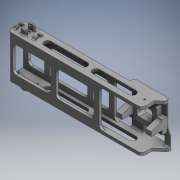
# Autodesk Inventor part: Arm Bottom Left
Saved by Autodesk Inventor 2020.5 (Build 245400000, 400)
## iProperties
Created: 2023-03-21
Part Number: Arm Bottom Left
Material: Generic
Document SubType Name: Modeling
Designer: Wes
Density: 1 g/cm^3
Appearance: Default
Author: Wes
Autodesk Inventor part; units mm, degrees
ref_plane "YZ Plane" through (0, 0, 0) normal (1, 0, 0) x (0, 1, 0)
ref_plane "XZ Plane" through (0, 0, 0) normal (0, 1, 0) x (-1, 0, 0)
ref_plane "XY Plane" through (0, 0, 0) normal (0, 0, 1) x (1, 0, 0)
sketch "Base" plane through (0, 0, 0) normal (0, 0, 1) x (1, 0, 0)
  line L0 (0, 0) -> (-30, 0)
  line L1 (-30, 0) -> (-30, 230)
  line L2 (-30, 230) -> (0, 230)
  line L3 (0, 230) -> (0, 0)
  dimension "d0" = 30
  dimension "d1" = 230
  constraints: 8 end point, 2 parallel, 1 horizontal, 1 perpendicular
  measures "d0" distance of L1.end L2.end
  measures "d1" distance of L0.end L1.end
extrude "Extrusion1" add sketch "Base" along normal blind 5
sketch "Axle Screw Countersink" plane through (0, 0, 5) normal (0, 0, 1) x (1, 0, 0)
  line L0 (-15, 0) -> (-15, 20) construction
  circle A0 centre (-15, 20) radius 3.15
  dimension "d4" = 20
  dimension "d58" = 6.3
  constraints: 2 end point, 1 centre point, 1 coincident, 1 vertical
  measures "d4" distance of L0.start L0.end
  measures "d58" diameter of A0
extrude "Extrusion2" cut sketch "Axle Screw Countersink" against normal blind 1.2
sketch "Motor Arm Center Fitting" plane through (0, 0, 5) normal (0, 0, 1) x (1, 0, 0)
  line L0 (-19.393, 15.95) -> (-19.393, 24.05) construction
  arc A0 (-19.393, 24.05) -> (-19.393, 15.95) centre (-15, 20) ccw
  line L1 (-19.393, 15.95) -> (-21.231, 14.2554)
  line L2 (-19.393, 24.05) -> (-21.231, 25.7446)
  line L3 (-15, 8.3504) -> (-15, 30.6989) construction
  arc A1 (-21.231, 25.7446) -> (-21.231, 14.2554) centre (-15, 20) ccw
  line L4 (-10.607, 15.95) -> (-10.607, 24.05) construction
  line L5 (-10.607, 15.95) -> (-19.393, 15.95) construction
  arc A2 (-10.607, 15.95) -> (-10.607, 24.05) centre (-15, 20) ccw
  line L6 (-10.607, 15.95) -> (-8.769, 14.2554)
  line L7 (-10.607, 24.05) -> (-8.769, 25.7446)
  arc A3 (-8.769, 14.2554) -> (-8.769, 25.7446) centre (-15, 20) ccw
  circle A4 centre (-15, 20) radius 5.975 construction
  point P0 (0, 0)
  point P1 (-15, 20)
  dimension "d18" = 11.95
  dimension "d19" = 8.1
  dimension "d20" = 8.1
  dimension "d21" = 2.5
  dimension "d22" = 2.5
  constraints: 16 end point, 12 point on circle, 5 centre point, 2 line through centre, 2 symmetric about line, 2 vertical, 1 concentric, 1 perpendicular, 2 other
  measures "d18" diameter of A4
  measures "d19" distance of L5.start L4.end
  measures "d20" distance of L5.end L0.end
  measures "d21" distance of L5.end L1.end
  measures "d22" distance of L0.end L2.end
extrude "Extrusion3" add sketch "Motor Arm Center Fitting" along normal blind 5
sketch "Motor Rotation Support" plane through (0, 0, 10) normal (0, 0, 1) x (1, 0, 0)
  line L0 (-20.975, 20) -> (-21.775, 20) construction
  circle A0 centre (-15, 20) radius 6.775 construction
  arc A1 (-19.9811, 24.5923) -> (-19.9811, 15.4077) centre (-15, 20) ccw
  line L1 (-21.775, 20) -> (-23.775, 20) construction
  circle A2 centre (-15, 20) radius 8.775 construction
  arc A3 (-21.4516, 25.9479) -> (-21.4516, 14.0521) centre (-15, 20) ccw
  line L2 (-21.4516, 14.0521) -> (-19.9811, 15.4077)
  line L3 (-19.9811, 24.5923) -> (-21.4516, 25.9479)
  line L4 (-15, 8.5295) -> (-15, 32.0479) construction
  line L5 (-8.5484, 14.0521) -> (-10.0189, 15.4077)
  arc A4 (-8.5484, 14.0521) -> (-8.5484, 25.9479) centre (-15, 20) ccw
  arc A5 (-10.0189, 15.4077) -> (-10.0189, 24.5923) centre (-15, 20) ccw
  line L6 (-10.0189, 24.5923) -> (-8.5484, 25.9479)
  point P0 (0, 0)
  point P1 (-21.231, 14.2554)
  point P2 (-21.231, 25.7446)
  dimension "d25" = 0.8
  dimension "d26" = 2
  constraints: 16 point on circle, 14 end point, 6 centre point, 4 symmetric about line, 2 coincident, 2 horizontal, 1 concentric, 1 vertical, 2 other
  measures "d25" distance of L0.start L0.end
  measures "d26" distance of L0.end L1.end
extrude "Extrusion4" add sketch "Motor Rotation Support" along normal blind 3.35
sketch "Motor Arm Screw Holes" plane through (0, 0, 5) normal (0, 0, 1) x (1, 0, 0)
  line L0 (-15, 20) -> (-15, 37.1) construction
  line L1 (-15, 20) -> (-15, 2.9) construction
  line L2 (-15, 20) -> (-15, 4.2) construction
  line L3 (-15, 20) -> (-15, 35.8) construction
  line L4 (-15, 4.2) -> (-15, 2.9) construction
  line L5 (-15, 35.8) -> (-15, 37.1) construction
  circle A0 centre (-15, 36.45) radius 1.175
  circle A1 centre (-15, 3.55) radius 1.175
  point P0 (0, 0)
  dimension "d59" = 34.2
  dimension "d60" = 31.6
  dimension "d61" = 2.35
  dimension "d62" = 2.35
  constraints: 12 end point, 3 vertical, 2 centre point, 2 midpoint, 2 point on line, 1 coincident, 1 collinear
  measures "d59" distance of L0.end L1.end
  measures "d60" distance of L3.end L2.end
  measures "d61" diameter of A0
  measures "d62" diameter of A1
extrude "Extrusion5" cut sketch "Motor Arm Screw Holes" against normal through all
sketch "Motor Arm Support" plane through (0, 0, 5) normal (0, 0, 1) x (1, 0, 0)
  line L0 (-15, 2.375) -> (-15, 6.875) construction
  line L1 (-15, 6.875) -> (-11.875, 6.875) construction
  line L2 (-15, 6.875) -> (-18.125, 6.875) construction
  line L3 (-15, 3.55) -> (-12.2, 3.55) construction
  line L4 (-15, 3.55) -> (-12.2, 3.55) construction
  line L5 (-15, 3.55) -> (-17.8, 3.55) construction
  line L6 (-15, 3.55) -> (-12.2, 3.55) construction
  line L7 (-18.125, 6.875) -> (-17.8, 3.55)
  line L8 (-17.8, 3.55) -> (-19.7905, 3.3554)
  line L9 (-19.7905, 3.3554) -> (-20.1155, 6.6804)
  line L10 (-20.1155, 6.6804) -> (-18.125, 6.875)
  line L11 (-11.875, 6.875) -> (-12.2, 3.55)
  line L12 (-12.2, 3.55) -> (-10.2095, 3.3554)
  line L13 (-9.8845, 6.6804) -> (-11.875, 6.875)
  line L14 (-10.2095, 3.3554) -> (-9.8845, 6.6804)
  line L15 (-17.8, 3.55) -> (-17.6054, 1.5595)
  line L16 (-17.6054, 1.5595) -> (-19.596, 1.3649)
  line L17 (-19.596, 1.3649) -> (-19.7905, 3.3554)
  line L18 (-12.2, 3.55) -> (-12.3946, 1.5595)
  line L19 (-12.3946, 1.5595) -> (-10.404, 1.3649)
  line L20 (-10.404, 1.3649) -> (-10.2095, 3.3554)
  arc A0 (-10.607, 15.95) -> (-10.607, 24.05) centre (-15, 20) ccw construction
  line L21 (-9.025, 20) -> (-20.975, 20) construction
  arc A1 (-19.393, 24.05) -> (-19.393, 15.95) centre (-15, 20) ccw construction
  line L22 (-15, 33.125) -> (-11.875, 33.125) construction
  line L23 (-15, 33.125) -> (-18.125, 33.125) construction
  line L24 (-11.875, 33.125) -> (-12.2, 36.45)
  line L25 (-10.2095, 36.6446) -> (-9.8845, 33.3196)
  line L26 (-9.8845, 33.3196) -> (-11.875, 33.125)
  line L27 (-18.125, 33.125) -> (-17.8, 36.45)
  line L28 (-19.7905, 36.6446) -> (-20.1155, 33.3196)
  line L29 (-20.1155, 33.3196) -> (-18.125, 33.125)
  line L30 (-17.8, 36.45) -> (-19.7905, 36.6446)
  line L31 (-15, 37.625) -> (-15, 33.125) construction
  line L32 (-15, 36.45) -> (-12.2, 36.45) construction
  line L33 (-15, 36.45) -> (-12.2, 36.45) construction
  line L34 (-15, 36.45) -> (-17.8, 36.45) construction
  line L35 (-15, 36.45) -> (-12.2, 36.45) construction
  line L36 (-19.596, 38.6351) -> (-19.7905, 36.6446)
  line L37 (-17.6054, 38.4405) -> (-19.596, 38.6351)
  line L38 (-17.8, 36.45) -> (-17.6054, 38.4405)
  line L39 (-12.2, 36.45) -> (-12.3946, 38.4405)
  line L40 (-12.2, 36.45) -> (-10.2095, 36.6446)
  line L41 (-10.404, 38.6351) -> (-10.2095, 36.6446)
  line L42 (-12.3946, 38.4405) -> (-10.404, 38.6351)
  point P0 (0, 0)
  dimension "d63" = 4.5
  dimension "d64" = 6.25
  dimension "d65" = 5.6
  dimension "d66" = 2
  dimension "d67" = 2
  constraints: 86 end point, 22 symmetric about line, 7 horizontal, 5 perpendicular, 2 collinear, 2 point on circle, 1 vertical
  measures "d63" distance of L0.start L1.start
  measures "d64" distance of L2.end L1.end
  measures "d65" distance of L7.end L3.end
  measures "d66" distance of L7.end L9.start
  measures "d67" distance of L7.end L16.start
extrude "Extrusion6" add sketch "Motor Arm Support" along normal blind 3
draft "FaceDraft1" angle 28 pull direction (0, 0, 1) faces at (-10.2309, 3.1368, 6) (-10.0577, 35.0914, 6) fixed edges at (-10.1443, 4.0227, 8) (-10.1443, 35.9773, 8)
draft "FaceDraft2" angle 28 pull direction (0, 0, 1) faces at (-19.9423, 4.9086, 6) (-19.7691, 36.8632, 6) fixed edges at (-19.8557, 4.0227, 8) (-19.8557, 35.9773, 8)
sketch "Axle Hole" plane through (0, 0, 5) normal (0, 0, 1) x (1, 0, 0)
  line L0 (0, 230) -> (-30, 230) construction
  line L1 (-15, 230) -> (-15, 220) construction
  circle A0 centre (-15, 220) radius 1.5
  point P0 (0, 0)
  dimension "d73" = 10
  dimension "d74" = 3
  constraints: 2 end point, 1 centre point, 1 coincident, 1 midpoint, 1 vertical
  measures "d73" distance of L1.start L1.end
  measures "d74" diameter of A0
extrude "Extrusion7" cut sketch "Axle Hole" against normal through all
sketch "Motor Backplate Offset" plane through (0, 0, 0) normal (0, 0, -1) x (-1, 0, 0)
  circle A0 centre (15, 220) radius 1.5 construction
  line L0 (15, 220) -> (15, 180) construction
  line L1 (15, 220) -> (15, 240) construction
  line L2 (30, 240) -> (33.5, 240)
  line L3 (33.5, 240) -> (33.5, 180)
  line L4 (33.5, 180) -> (30, 180)
  line L5 (30, 180) -> (30, 240)
  point P0 (0, 0)
  dimension "d77" = 40
  dimension "d78" = 20
  dimension "d83" = 3.5
  dimension "d84" = 60
  constraints: 12 end point, 2 parallel, 2 vertical, 1 horizontal, 1 perpendicular
  measures "d77" distance of L0.start L0.end
  measures "d78" distance of L0.start L1.end
  measures "d83" distance of L3.end L4.end
  measures "d84" distance of L0.end L1.end
extrude "Extrusion8" add sketch "Motor Backplate Offset" against normal up to surface (5 mm away)
sketch "Motor Backplate" plane through (0, 0, 0) normal (0, 0, -1) x (-1, 0, 0)
  line L0 (33.5, 180) -> (33.5, 240) projected
  line L1 (33.5, 240) -> (37.5, 240)
  line L2 (37.5, 240) -> (37.5, 180)
  line L3 (37.5, 180) -> (33.5, 180)
  line L4 (33.5, 180) -> (33.5, 240)
  point P0 (0, 0)
  dimension "d85" = 4
  constraints: 8 end point, 2 parallel, 1 horizontal, 1 perpendicular
  measures "d85" distance of L2.end L3.end
extrude "Extrusion9" add sketch "Motor Backplate" along normal blind 63 and the other way blind 5
sketch "Axle Reference" plane through (0, 0, 0) normal (0, 0, -1) x (-1, 0, 0)
  circle A0 centre (15, 220) radius 1.5 construction
  line L0 (15, 220) -> (24.935, 220) construction
  point P0 (0, 0)
  dimension "d98" = 9.935
  constraints: 2 end point, 1 horizontal
  measures "d98" distance of L0.start L0.end
sketch "Motor Riser" plane through (-33.5, 180, 0) normal (1, 0, 0) x (0, 0, -1)
  line L0 (0, 30) -> (7, 30) construction
  line L1 (7, 30) -> (43, 30) construction
  line L2 (43, 60) -> (20, 60)
  line L3 (20, 60) -> (20, 0)
  line L4 (20, 0) -> (43, 0)
  line L5 (43, 0) -> (43, 60)
  line L6 (7, 30) -> (7, 51)
  line L7 (7, 30) -> (7, 9)
  line L8 (7, 51) -> (20, 51)
  line L9 (7, 9) -> (20, 9)
  line L10 (63, 0) -> (-5, 0) construction
  line L11 (0, 0) -> (0, 60) construction
  point P0 (0, -180)
  dimension "d90" = 7
  dimension "d92" = 36
  dimension "d93" = 23
  dimension "d94" = 60
  dimension "d97" = 42
  constraints: 22 end point, 4 perpendicular, 3 horizontal, 3 point on line, 2 parallel, 2 vertical, 1 midpoint
  measures "d90" distance of L0.start L0.end
  measures "d92" distance of L0.end L1.end
  measures "d93" distance of L4.end L3.end
  measures "d94" distance of L3.end L2.end
  measures "d97" distance of L7.end L6.end
extrude "Extrusion10" add sketch "Motor Riser" along normal up to surface (8.565 mm away)
sketch "Motor Attachment Towers" plane through (-24.935, 180, -43) normal (1, 0, 0) x (0, 0, -1)
  line L0 (0, 60) -> (0, 0) construction
  line L1 (0, 30) -> (-7, 30) construction
  line L2 (-7, 30) -> (-7, 9.8) construction
  line L3 (-7, 30) -> (-7, 50.2) construction
  line L4 (-7, 9.8) -> (-14.5, 9.8)
  line L5 (-14.5, 9.8) -> (-14.5, 0)
  line L6 (-14.5, 0) -> (-7, 0)
  line L7 (-7, 0) -> (-7, 9.8)
  line L8 (-48, 60) -> (20, 60) projected
  line L9 (-7, 50.2) -> (-14.5, 50.2)
  line L10 (-14.5, 50.2) -> (-14.5, 60)
  line L11 (-14.5, 60) -> (-7, 60)
  line L12 (-7, 60) -> (-7, 50.2)
  point P0 (-43, -180)
  point P1 (-7, 60)
  dimension "d101" = 7
  dimension "d102" = 20.2
  dimension "d104" = 40.4
  dimension "d105" = 7.5
  dimension "d106" = 9.8
  constraints: 22 end point, 4 parallel, 3 horizontal, 2 perpendicular, 2 vertical, 1 midpoint, 1 point on line
  measures "d101" distance of L1.start L1.end
  measures "d102" distance of L1.end L2.end
  measures "d104" distance of L3.end L2.end
  measures "d105" distance of L6.end L5.end
  measures "d106" distance of L5.end L4.end
extrude "Extrusion11" add sketch "Motor Attachment Towers" along normal blind 18.5
sketch "Motor Screw Holes" plane through (-24.935, 180, -36) normal (0, 0, -1) x (-1, 0, 0)
  circle A0 centre (-9.935, 40) radius 1.5 construction
  line L0 (-9.935, 40) -> (-9.935, 54.55) construction
  line L1 (-9.935, 40) -> (-9.935, 5.7) construction
  line L2 (-9.935, 5.7) -> (-14.845, 5.7) construction
  line L3 (-9.935, 5.7) -> (-5.025, 5.7) construction
  circle A1 centre (-14.845, 5.7) radius 1.275
  circle A2 centre (-5.025, 5.7) radius 1.275
  line L4 (0, 60) -> (0, 0) construction
  line L5 (0, 30) -> (-23.1179, 30) construction
  circle A3 centre (-14.845, 54.3) radius 1.275
  circle A4 centre (-5.025, 54.3) radius 1.275
  point P0 (-24.935, -180)
  dimension "d109" = 14.55
  dimension "d110" = 34.3
  dimension "d111" = 4.91
  dimension "d113" = 9.82
  dimension "d114" = 2.55
  dimension "d115" = 2.55
  constraints: 10 end point, 4 centre point, 3 horizontal, 2 coincident, 2 symmetric about line, 2 vertical, 1 midpoint, 2 other
  measures "d109" distance of L0.start L0.end
  measures "d110" distance of L0.start L1.end
  measures "d111" distance of L1.end L2.end
  measures "d113" distance of L3.end L2.end
  measures "d114" diameter of A1
  measures "d115" diameter of A2
extrude "Extrusion12" cut sketch "Motor Screw Holes" against normal blind 4
draft "FaceDraft3" angle 18 pull direction (1, 0, 0) faces at (-18.7683, 236.7333, -28.5) (-18.7683, 186.5333, -28.5) fixed edges at (-6.435, 235.1, -28.5) (-6.435, 184.9, -28.5)
ref_plane "Arm Clearance Offset Plane" through (-33.5, 180, -50) normal (0, 0, -1) x (-1, 0, 0)
sketch "Arm Clearance Cut" plane through (-33.5, 180, -50) normal (0, 0, -1) x (-1, 0, 0)
  circle A0 centre (-18.5, 40) radius 1.5 construction
  line L0 (-18.5, 40) -> (-0.8231, 30.6445) construction
  line L1 (-14.6733, 21.324) -> (-88.9165, 60.6172)
  line L2 (-92.245, 71.4302) -> (-85.6962, 83.804)
  line L3 (-74.8832, 87.1326) -> (-0.64, 47.8395)
  line L4 (2.6886, 37.0265) -> (-3.8603, 24.6526)
  arc A1 (-92.245, 71.4302) -> (-88.9165, 60.6172) centre (-85.1743, 67.688) ccw
  arc A2 (-74.8832, 87.1326) -> (-85.6962, 83.804) centre (-78.6254, 80.0618) ccw
  arc A3 (-14.6733, 21.324) -> (-3.8603, 24.6526) centre (-10.9311, 28.3948) ccw
  arc A4 (2.6886, 37.0265) -> (-0.64, 47.8395) centre (-4.3822, 40.7687) ccw
  line L5 (-8.565, 9) -> (-8.565, 51) construction
  line L6 (-8.565, 19.2396) -> (4, 19.2396) construction
  line L7 (4, 60) -> (4, 0) construction
  line L8 (0, 51) -> (0, 60) construction
  line L9 (0, 60) -> (0, 56) construction
  line L10 (0, 9) -> (0, 51) projected
  line L11 (0, 19.2396) -> (4, 19.2396)
  line L12 (4, 19.2396) -> (4, 56)
  line L13 (4, 56) -> (0, 56)
  line L14 (0, 56) -> (0, 19.2396)
  point P0 (-33.5, -180)
  point P1 (-81.954, 90.8748)
  point P2 (-95.9872, 64.3594)
  point P3 (6.4308, 44.0973)
  dimension "d119" = 20
  dimension "d120" = 100
  dimension "d121" = 30
  dimension "d122" = 8
  dimension "d124" = 4
  constraints: 22 end point, 12 point on line, 8 point on circle, 8 tangent, 4 centre point, 4 parallel, 3 equal radius, 2 horizontal, 2 perpendicular
  measures "d119" distance of A0.centre L0.end
  measures "d120" distance of point (-81.954, 90.875) point (6.431, 44.097)
  measures "d121" distance of point (-95.987, 64.359) point (-81.954, 90.875)
  measures "d122" radius of A1
  measures "d124" distance of L8.end L9.end
extrude "Extrusion13" cut sketch "Arm Clearance Cut" along normal up to surface (13 mm away) contours L10 A4 L4 | L4 A4 L10 L14 L13 L12 L11
sketch "Connector Support" plane through (-33.5, 180, -50) normal (0, 0, -1) x (-1, 0, 0)
  line L0 (4, 60) -> (0, 60) projected
  line L1 (4, 60) -> (0, 60)
  line L2 (0, 60) -> (0, 65)
  line L3 (0, 65) -> (4, 65)
  line L4 (4, 65) -> (4, 60)
  point P0 (-33.5, -180)
  dimension "d127" = 5
  constraints: 8 end point, 2 parallel, 1 horizontal, 1 perpendicular
  measures "d127" distance of L1.end L2.end
extrude "Extrusion14" add sketch "Connector Support" along normal blind 13 and the other way blind 4
sketch "Sketch18" plane through (0, 0, -63) normal (0, 0, -1) x (-1, 0, 0)
  line L0 (0, 0) -> (0, 230) projected
  line L1 (0, 0) -> (30, 0)
  line L2 (30, 0) -> (30, 230)
  line L3 (30, 230) -> (0, 230)
  line L4 (0, 230) -> (0, 0)
  line L5 (33.5, 180) -> (24.935, 180) projected
  line L6 (37.5, 245) -> (37.5, 240) projected
  line L7 (30, 180) -> (37.5, 180)
  line L8 (37.5, 180) -> (37.5, 245)
  line L9 (37.5, 245) -> (30, 245)
  line L10 (30, 245) -> (30, 180)
  constraints: 16 end point, 4 parallel, 2 horizontal, 2 perpendicular, 2 point on line
extrude "Extrusion17" add sketch "Sketch18" along normal blind 5
ref_plane "Work Plane2" through (0, 0, -31.5) normal (0, 0, -1) x (-1, 0, 0)
mirror "Mirror1" about plane through (0, 0, -31.5) normal (0, 0, -1) of "Extrusion5", "Extrusion6", "Extrusion4", "Extrusion3", "Extrusion2", "FaceDraft1", "FaceDraft2"
draft "FaceDraft4" angle 40 pull direction (0, 1, 0) faces at (-30, 236.6667, 1.6667) (-30, 240, -64.6667) fixed edges at (-30, 240, 2.5) (-30, 245, -65.5)
draft "FaceDraft5" angle 65 pull direction (0, 1, 0) faces at (-34.8333, 243.3333, -46) fixed edges at (-35.5, 245, -46)
sketch "Sketch20" plane through (-24.935, 180, -43) normal (1, 0, 0) x (0, 0, -1)
  line L0 (-36, 9) -> (-36, 51) construction
  line L1 (-36, 30) -> (-28, 30) construction
  line L2 (0, 60) -> (0, 0) construction
  line L3 (0, 30) -> (-8, 30) construction
  line L4 (-7, 50.2) -> (-20.511, 50.2) construction
  line L5 (-20.511, 50.2) -> (-20.511, 43.2) construction
  line L6 (-20.511, 9.8) -> (-14.5, 9.8) construction
  line L7 (-20.511, 9.8) -> (-20.511, 16.8) construction
  line L8 (-24, 43.2) -> (-12, 43.2)
  line L9 (-8, 39.2) -> (-8, 20.8)
  line L10 (-12, 16.8) -> (-24, 16.8)
  line L11 (-28, 20.8) -> (-28, 39.2)
  arc A0 (-24, 43.2) -> (-28, 39.2) centre (-24, 39.2) ccw
  arc A1 (-8, 39.2) -> (-12, 43.2) centre (-12, 39.2) ccw
  arc A2 (-28, 20.8) -> (-24, 16.8) centre (-24, 20.8) ccw
  arc A3 (-12, 16.8) -> (-8, 20.8) centre (-12, 20.8) ccw
  point P0 (-43, -180)
  dimension "d146" = 8
  dimension "d147" = 8
  dimension "d148" = 7
  dimension "d149" = 7
  dimension "d150" = 4
  constraints: 16 end point, 8 point on circle, 8 tangent, 4 centre point, 3 equal radius, 3 horizontal, 2 midpoint, 2 parallel, 2 vertical, 1 perpendicular
  measures "d146" distance of L1.start L1.end
  measures "d147" distance of L3.start L3.end
  measures "d148" distance of L4.end L5.end
  measures "d149" distance of L6.start L7.end
  measures "d150" radius of A0
extrude "Extrusion18" cut sketch "Sketch20" against normal up to surface (12.565 mm away)
sketch "Sketch21" plane through (0, 0, 0) normal (1, 0, 0) x (0, 0, -1)
  line L0 (35.9641, 180) -> (35.9641, 157) construction
  line L1 (35.9641, 180) -> (58.9641, 180) construction
  line L2 (0, 0) -> (-5, 0) projected
  line L3 (63, 0) -> (63, 180) projected
  line L4 (0, 0) -> (63, 0)
  line L5 (63, 0) -> (63, 157)
  line L6 (63, 157) -> (0, 157)
  line L7 (0, 157) -> (0, 0)
  line L8 (0, 180) -> (0, 0) construction
  line L9 (0, 75.2833) -> (9, 75.2833) construction
  line L10 (63, 75.2833) -> (54, 75.2833) construction
  line L11 (38.8064, 0) -> (38.8064, 9) construction
  line L12 (38.8064, 157) -> (38.8064, 148) construction
  line L13 (9, 9) -> (54, 9)
  line L14 (54, 9) -> (54, 148)
  line L15 (54, 148) -> (9, 148)
  line L16 (9, 148) -> (9, 9)
  line L17 (9, 74) -> (54, 74)
  line L18 (54, 74) -> (54, 83)
  line L19 (54, 83) -> (9, 83)
  line L20 (9, 83) -> (9, 74)
  line L21 (9, 74) -> (54, 83) construction
  line L22 (54, 74) -> (9, 83) construction
  point P0 (31.5, 78.5)
  dimension "d153" = 23
  dimension "d157" = 9
  dimension "d158" = 9
  dimension "d159" = 9
  dimension "d160" = 9
  dimension "d161" = 9
  constraints: 40 end point, 6 parallel, 6 perpendicular, 6 point on line, 4 horizontal, 3 vertical, 2 midpoint
  measures "d153" distance of L0.start L0.end
  measures "d157" distance of L9.start L9.end
  measures "d158" distance of L10.start L10.end
  measures "d159" distance of L11.start L11.end
  measures "d160" distance of L12.start L12.end
  measures "d161" distance of L18.end L17.end
extrude "Extrusion19" add sketch "Sketch21" against normal blind 4 contours L4 L7 L6 L3 | L16 L19 L14 L17
sketch "Sketch22" plane through (-30, 0, -63) normal (-1, 0, 0) x (0, 0, 1)
  line L0 (0, 0) -> (0, 180) projected
  line L1 (0, 157) -> (63, 157) projected
  line L2 (0, 0) -> (63, 0)
  line L3 (63, 0) -> (63, 157)
  line L4 (63, 157) -> (0, 157)
  line L5 (0, 157) -> (0, 0)
  line L6 (9, 9) -> (54, 9) projected
  line L7 (54, 148) -> (54, 83) projected
  line L8 (9, 9) -> (54, 9)
  line L9 (54, 9) -> (54, 148)
  line L10 (54, 148) -> (9, 148)
  line L11 (9, 148) -> (9, 9)
  line L12 (54, 74) -> (54, 9) projected
  line L13 (9, 37) -> (54, 37)
  line L14 (54, 37) -> (54, 46)
  line L15 (54, 46) -> (9, 46)
  line L16 (9, 46) -> (9, 37)
  line L17 (9, 37) -> (54, 46) construction
  line L18 (54, 37) -> (9, 46) construction
  line L19 (9, 111) -> (54, 111)
  line L20 (54, 111) -> (54, 120)
  line L21 (54, 120) -> (9, 120)
  line L22 (9, 120) -> (9, 111)
  line L23 (9, 111) -> (54, 120) construction
  line L24 (54, 111) -> (9, 120) construction
  point P0 (31.5, 41.5)
  point P1 (31.5, 115.5)
  dimension "d164" = 9
  dimension "d165" = 9
  constraints: 40 end point, 8 parallel, 4 horizontal, 4 midpoint, 4 perpendicular, 2 point on line
  measures "d164" distance of L14.end L13.end
  measures "d165" distance of L20.end L19.end
extrude "Extrusion20" add sketch "Sketch22" against normal blind 4 contours L0 L1 L3 L2 | L11 L15 L9 L13 | L11 L21 L7 L19
sketch "Sketch24" plane through (0, 0, 5) normal (0, 0, 1) x (1, 0, 0)
  line L0 (0, 0) -> (0, 230) construction
  line L1 (0, 123.8121) -> (-9, 123.8121) construction
  line L2 (-30, 180) -> (-30, 0) construction
  line L3 (-30, 123.8121) -> (-21, 123.8121) construction
  line L4 (-30, 123.8121) -> (-21, 123.8121) construction
  circle A0 centre (-15, 220) radius 1.5 construction
  line L5 (-15, 220) -> (-15, 205) construction
  circle A1 centre (-15, 36.45) radius 1.175 construction
  line L6 (-15, 36.45) -> (-15, 47.45) construction
  line L7 (-9, 205) -> (-21, 205)
  line L8 (-21, 205) -> (-21, 47.45)
  line L9 (-21, 47.45) -> (-9, 47.45)
  line L10 (-9, 47.45) -> (-9, 205)
  line L11 (-9, 130.725) -> (-21, 130.725)
  line L12 (-21, 130.725) -> (-21, 121.725)
  line L13 (-21, 121.725) -> (-9, 121.725)
  line L14 (-9, 121.725) -> (-9, 130.725)
  line L15 (-9, 130.725) -> (-21, 121.725) construction
  line L16 (-21, 130.725) -> (-9, 121.725) construction
  point P0 (-15, 126.225)
  dimension "d180" = 9
  dimension "d182" = 9
  dimension "d184" = 15
  dimension "d185" = 11
  dimension "d186" = 9
  constraints: 30 end point, 5 horizontal, 4 parallel, 3 point on line, 2 midpoint, 2 perpendicular, 2 vertical, 1 collinear
  measures "d180" distance of L1.start L1.end
  measures "d182" distance of L3.start L3.end
  measures "d184" distance of L5.start L5.end
  measures "d185" distance of L6.start L6.end
  measures "d186" distance of L12.end L11.end
extrude "Extrusion22" cut sketch "Sketch24" against normal up to surface (5 mm away) contours L10 L11 L8 L7 | L10 L9 L8 L13
mirror "Mirror2" about plane through (0, 0, -31.5) normal (0, 0, -1) of "Extrusion22"
fillet "Fillet1" radius 2 6 edges at (-23.475, 20, 5) (-6.525, 20, 5) (-8.225, 20, 10) (-21.775, 20, 10) (-6.525, 20, -68) (-23.475, 20, -68)
fillet "Fillet2" radius 6 39 edges at (-2, 148, -9) (-28, 148, -9) (-2, 148, -54) (-28, 148, -54) (-28, 120, -9) (-28, 120, -54) (-2, 83, -54) (-2, 83, -9) (-2, 74, -9) (-2, 74, -54) (-2, 9, -9) (-28, 9, -9) (-28, 9, -54) (-2, 9, -54) (-28, 46, -54) (-28, 111, -9) (-28, 46, -9) (-28, 37, -9) (-28, 111, -54) (-9, 130.725, 2.5) (-21, 130.725, 2.5) (-21, 47.45, 2.5) (-21, 130.725, -65.5) (-21, 47.45, -65.5) (-21, 121.725, -65.5) (-21, 121.725, 2.5) (-21, 205, 2.5) (-21, 205, -65.5) (-9, 121.725, -65.5) (-9, 205, -65.5) (-9, 205, 2.5) (-9, 47.45, 2.5) (-9, 47.45, -65.5) (-9, 130.725, -65.5) (-9, 121.725, 2.5) (-28, 157, 0) (-2, 157, 0) (-28, 157, -63) (-2, 157, -63)
fillet "Fillet3" radius 3 24 edges at (-37.5, 245, -57) (-37.5, 242.5, -40.6387) (-37.5, 240, -15.1387) (-30, 240, 2.5) (-30, 245, -65.5) (-21.609, 230, 2.5) (-17.4135, 230, -65.5) (-37.5, 180, -31.5) (-30, 180, 2.5) (-30, 180, -65.5) (-29.2175, 189, -7) (-29.2175, 231, -7) (-24.935, 235.1, -22.489) (-24.935, 184.9, -22.489) (-33.5, 240.5, -63) (-33.5, 189.6198, -63) (-8.5567, 36.1325, -68) (-8.5567, 3.8675, -68) (-21.4433, 3.8675, -68) (-21.4433, 36.1325, -68) (-8.5567, 36.1325, 5) (-21.4433, 36.1325, 5) (-8.5567, 3.8675, 5) (-21.4433, 3.8675, 5)
fillet "Fillet4" radius 7 4 edges at (0, 0, -31.5) (-30, 0, -31.5) (0, 230, 2.5) (0, 230, -65.5)
body "Solid1"
